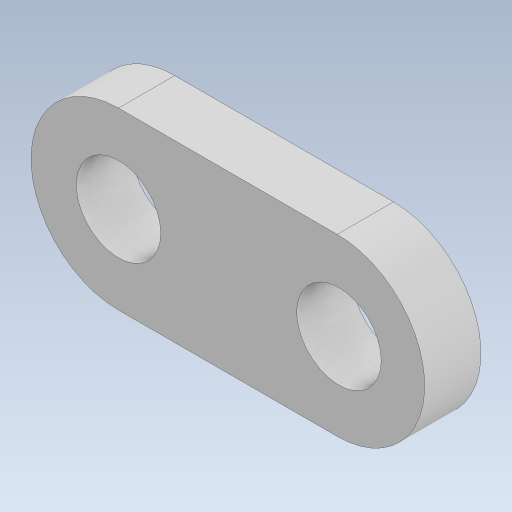
# Autodesk Inventor part: R3
Saved by Autodesk Inventor 2023 (Build 270158000, 158)
## iProperties
Created: 2022-09-16
Part Number: R3
Material: Generic
Document SubType Name: Modeling
Designer: Dave
Density: 1 g/cm^3
Appearance: Default
Author: Dave
## iProperties of the stored document R3_3DPrint.ipt
Created: 2022-09-16
Part Number: R3_3DPrint
Material: Generic
Document SubType Name: Modeling
Designer: Dave
Density: 1 g/cm^3
Appearance: Default
Author: Dave
Autodesk Inventor part; units mm, degrees
ref_plane "YZ Plane" through (0, 0, 0) normal (1, 0, 0) x (0, 1, 0)
ref_plane "XZ Plane" through (0, 0, 0) normal (0, 1, 0) x (-1, 0, 0)
ref_plane "XY Plane" through (0, 0, 0) normal (0, 0, 1) x (1, 0, 0)
sketch "Sketch2" plane through (0, 0, 0) normal (0, 1, 0) x (-1, 0, 0)
  line L0 (0, -4.5) -> (-31.5, -4.5)
  line L1 (-31.5, -4.5) -> (-31.5, 0)
  line L2 (-31.5, 0) -> (0, 0)
  line L3 (0, 0) -> (0, -4.5)
  line L4 (-7, -4.5) -> (-7, 0) construction
  line L5 (-24.5, 0) -> (-24.5, -4.5) construction
  point P0 (-7, -2.25)
  point P1 (-24.5, -2.25)
  dimension "d7" = 17.5
  dimension "d8" = 4.5
  dimension "d9" = 7
  dimension "d11" = 7
  constraints: 12 end point, 4 point on line, 3 perpendicular, 2 midpoint, 2 parallel, 1 coincident, 1 horizontal
  measures "d7" distance of point (-7, -2.25) point (-24.5, -2.25)
  measures "d8" distance between parallel lines of L0 L2
  measures "d9" distance between parallel lines of L3 L4
  measures "d11" distance between parallel lines of L5 L1
extrude "Extrusion1" add sketch "Sketch2" along normal blind 14
sketch "Sketch3" plane through (0, 0, 0) normal (0, 0, 1) x (1, 0, 0)
  line L0 (31.5, 0) -> (31.5, 14) projected
  line L1 (0, 0) -> (0, 14) projected
  point P0 (7, 7)
  point P1 (24.64, 7)
  point P2 (31.5, 7)
  dimension "d14" = 17.64
  dimension "d15" = 7
  constraints: 2 horizontal alignment, 1 midpoint
  measures "d14" distance of point (24.64, 7) point (7, 7)
  measures "d15" distance from line of L1 point (7, 7)
hole "Hole1" at (7, 7, 0) at (24.64, 7, 0) direction (0, 0, -1) diameter 6.756 end through all clearance for "Flat Head Machine Screw (82)" size "1/4" standard "Ansi Unified Screw Threads"
fillet "Fillet1" radius 7 4 edges at (0, 14, -2.25) (0, 0, -2.25) (31.5, 0, -2.25) (31.5, 14, -2.25)
body "Solid1"
